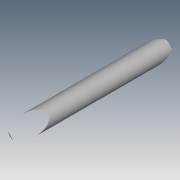
# Autodesk Inventor part: shaft5
Saved by Autodesk Inventor 2015 (Build 190159000, 159)
## iProperties
Created: 2014-08-31
Part Number: shaft5
Material: Generic
Document SubType Name: Modeling
Designer: shohei
Density: 1 g/cm^3
Appearance: Default
Mass: 6.28319 g
Surface Area: 26.7035 cm^2
Volume: 6.28319 cm^3
Author: shohei
Autodesk Inventor part; units mm, degrees
ref_plane "YZ Plane" through (0, 0, 0) normal (1, 0, 0) x (0, 1, 0)
ref_plane "XZ Plane" through (0, 0, 0) normal (0, 1, 0) x (-1, 0, 0)
ref_plane "XY Plane" through (0, 0, 0) normal (0, 0, 1) x (1, 0, 0)
sketch "Sketch1" plane through (0, 0, 0) normal (0, 1, 0) x (-1, 0, 0)
  circle A0 centre (0, 0) radius 5
  dimension "d0" = 10
  constraints: 1 centre point, 1 coincident
  measures "d0" diameter of A0
extrude "Extrusion1" add sketch "Sketch1" along normal blind 80
body "Solid1"
